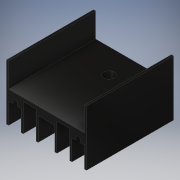
# Autodesk Inventor part: Kühlkörper
Saved by Autodesk Inventor 2017 SP1 (Build 210196100, 196)
## iProperties
Part Number: Kühlkörper
Material: Generisch
Document SubType Name: Modeling
Designer: Alex
Density: 1 g/cm^3
Appearance: Vorgabe
Author: Alex
Autodesk Inventor part; units mm, degrees
ref_plane "YZ Plane" through (0, 0, 0) normal (1, 0, 0) x (0, 1, 0)
ref_plane "XZ Plane" through (0, 0, 0) normal (0, 1, 0) x (-1, 0, 0)
ref_plane "XY Plane" through (0, 0, 0) normal (0, 0, 1) x (1, 0, 0)
sketch "Skizze1" plane through (0, 0, 0) normal (0, 1, 0) x (-1, 0, 0)
  line L0 (0, 16) -> (0, 0)
  line L1 (0, 16) -> (-0.6, 16)
  line L2 (-0.6, 16) -> (-0.6, 9)
  line L3 (0, 0) -> (-0.6, 0)
  line L4 (0, 0) -> (0.6, 0) construction
  line L5 (-0.6, 0) -> (-0.6, 6)
  line L6 (-4.2, 6) -> (-3.2, 6)
  line L7 (-3.2, 6) -> (-3.2, 6.5)
  arc A0 (-1.7, 6.5) -> (-3.2, 6.5) centre (-2.45, 6.5) ccw
  line L8 (-1.7, 6.5) -> (-1.7, 6)
  line L9 (-1.7, 6) -> (-0.6, 6)
  line L10 (-11.5, 23.3819) -> (-11.5, -15) construction
  line L11 (-4.2, 6) -> (-4.2, 0)
  line L12 (-4.2, 0) -> (-4.8, 0)
  line L13 (-4.8, 0) -> (-4.8, 8)
  line L14 (-4.8, 8) -> (-8.5, 8)
  line L15 (-0.6, 9) -> (-11.5, 9)
  line L16 (-8.5, 8) -> (-8.5, 0)
  line L17 (-8.5, 0) -> (-9.1, 0)
  line L18 (-9.1, 0) -> (-9.1, 6.7)
  line L19 (-9.1, 6.7) -> (-11.5, 6.7)
  line L20 (-23, 16) -> (-23, 0)
  line L21 (-23, 16) -> (-22.4, 16)
  line L22 (-22.4, 16) -> (-22.4, 9)
  line L23 (-23, 0) -> (-22.4, 0)
  line L24 (-23, 0) -> (-23.6, 0) construction
  line L25 (-22.4, 0) -> (-22.4, 6)
  line L26 (-19.8, 6) -> (-19.8, 6.5)
  line L27 (-18.8, 6) -> (-19.8, 6)
  arc A1 (-19.8, 6.5) -> (-21.3, 6.5) centre (-20.55, 6.5) ccw
  line L28 (-21.3, 6.5) -> (-21.3, 6)
  line L29 (-21.3, 6) -> (-22.4, 6)
  line L30 (-18.8, 6) -> (-18.8, 0)
  line L31 (-18.8, 0) -> (-18.2, 0)
  line L32 (-18.2, 0) -> (-18.2, 8)
  line L33 (-18.2, 8) -> (-14.5, 8)
  line L34 (-22.4, 9) -> (-11.5, 9)
  line L35 (-14.5, 8) -> (-14.5, 0)
  line L36 (-14.5, 0) -> (-13.9, 0)
  line L37 (-13.9, 0) -> (-13.9, 6.7)
  line L38 (-13.9, 6.7) -> (-11.5, 6.7)
  point P0 (0, 0)
  point P1 (-23, 0)
  dimension "d0" = 16
  dimension "d1" = 0.6
  dimension "d2" = 7
  dimension "d22" = 0.6
  dimension "d24" = 6
  dimension "d25" = 1
  dimension "d26" = 0.5
  dimension "d27" = 90
  dimension "d28" = 1.1
  dimension "d29" = 0.75
  dimension "d30" = 1.25
  dimension "d31" = 1.25
  dimension "d32" = 1.5
  dimension "d37" = 0.6
  dimension "d38" = 8
  dimension "d39" = 3.7
  dimension "d40" = 23
  dimension "d41" = 0.6
  dimension "d42" = 6.7
  dimension "d43" = 2.3
  constraints: 78 end point, 21 symmetric about line, 8 perpendicular, 7 vertical, 4 horizontal, 4 point on circle, 2 centre point, 2 coincident, 2 collinear, 2 point on line, 1 other
  measures "d0" distance of L0.start L0.end
  measures "d1" distance of L0.start L1.end
  measures "d2" distance of L1.end L2.end
  measures "d22" distance of L0.end L3.end
  measures "d24" distance of L3.end L5.end
  measures "d25" distance of L6.start L7.start
  measures "d26" distance of L7.start L7.end
  measures "d27" angle of L7 L6
  measures "d28" distance of L5.end L8.end
  measures "d29" radius of A0
  measures "d32" distance of L7.start L8.end
  measures "d37" distance of L11.end L12.end
  measures "d38" distance of L12.end L13.end
  measures "d39" distance of L13.end L14.end
  measures "d40" diameter of L0 L10
  measures "d41" distance of L16.end L17.end
  measures "d42" distance of L17.end L18.end
  measures "d43" distance between parallel lines of L19 L15
extrude "Extrusion1" add sketch "Skizze1" along normal blind 25
sketch "Skizze2" plane through (13.9, 0, 6.7) normal (0, 0, -1) x (-1, 0, 0)
  line L0 (0, 25) -> (4.8, 25) projected
  line L1 (0, 0) -> (0, 25) projected
  point P0 (13.9, 0)
  point P1 (2.4, 18)
  dimension "d46" = 7
  dimension "d47" = 2.4
  measures "d46" distance from line of point (2.4, 18) L0
  measures "d47" distance from line of L1 point (2.4, 18)
hole "Bohrung1" at (11.5, 18, 6.7) direction (0, 0, 1) diameter 3 end through all
